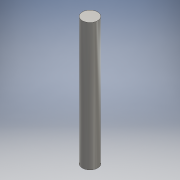
# Autodesk Inventor part: 平行ピン　φ1.2　長さ10
Saved by Autodesk Inventor 2016 (Build 200138000, 138)
## iProperties
Created: 2018-12-09
Part Number: 平行ピン　φ1.2　長さ10
Material: ステンレス鋼
Document SubType Name: Modeling
Designer: mozar
Density: 8 g/cm^3
Appearance: 半つや出し
Author: mozar
Autodesk Inventor part; units mm, degrees
ref_plane "YZ Plane" through (0, 0, 0) normal (1, 0, 0) x (0, 1, 0)
ref_plane "XZ Plane" through (0, 0, 0) normal (0, 1, 0) x (-1, 0, 0)
ref_plane "XY Plane" through (0, 0, 0) normal (0, 0, 1) x (1, 0, 0)
sketch "スケッチ1" plane through (0, 0, 0) normal (0, 0, 1) x (1, 0, 0)
  circle A0 centre (0, 0) radius 0.6
  dimension "d0" = 1.2
  constraints: 1 centre point, 1 coincident
  measures "d0" diameter of A0
extrude "押し出し1" add sketch "スケッチ1" along normal blind 10
